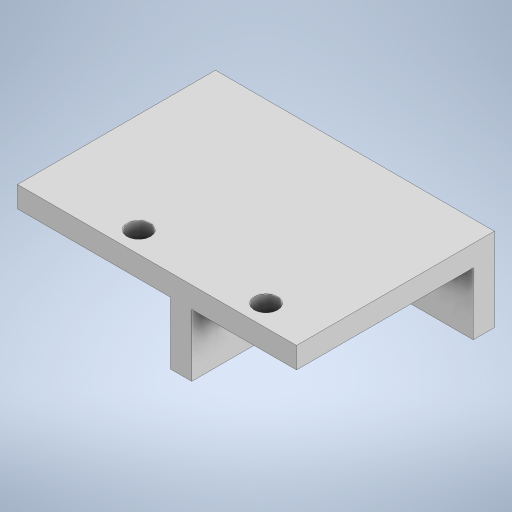
# Autodesk Inventor part: RatPelletBox_v02_holetest
Saved by Autodesk Inventor 2023.5 (Build 275446000, 446)
## iProperties
Created: 2025-06-19
Part Number: RatPelletBox_v02_holetest
Material: Generic
Document SubType Name: Modeling
Designer: Akramilab
Density: 1 g/cm^3
Appearance: Default
Author: Akramilab
Autodesk Inventor part; units mm, degrees
ref_plane "YZ Plane" through (0, 0, 0) normal (1, 0, 0) x (0, 1, 0)
ref_plane "XZ Plane" through (0, 0, 0) normal (0, 1, 0) x (-1, 0, 0)
ref_plane "XY Plane" through (0, 0, 0) normal (0, 0, 1) x (1, 0, 0)
sketch "Sketch1" plane through (0, 0, 0) normal (0, 0, 1) x (1, 0, 0)
  line L0 (-109, -87.5) -> (109, -87.5)
  line L1 (109, -87.5) -> (109, 87.5)
  line L2 (109, 87.5) -> (-109, 87.5)
  line L3 (-109, 87.5) -> (-109, -87.5)
  line L4 (-109, -87.5) -> (109, 87.5) construction
  line L5 (109, -87.5) -> (-109, 87.5) construction
  point P0 (0, 0)
  dimension "d0" = 218
  dimension "d1" = 175
  constraints: 12 end point, 2 midpoint, 2 parallel, 1 horizontal, 1 perpendicular
  measures "d0" distance of L1.end L2.end
  measures "d1" distance of L0.end L1.end
extrude "Extrusion1" add sketch "Sketch1" along normal blind 28
sketch "Sketch2" plane through (0, 0, 28) normal (0, 0, 1) x (1, 0, 0)
  line L0 (-106, 84.5) -> (-66, 84.5)
  line L1 (-66, 84.5) -> (-66, 44.5)
  line L2 (-66, 44.5) -> (-106, 44.5)
  line L3 (-106, 44.5) -> (-106, 84.5)
  line L4 (-106, 84.5) -> (-66, 44.5) construction
  line L5 (-66, 84.5) -> (-106, 44.5) construction
  line L6 (109, 87.5) -> (-109, 87.5) projected
  line L7 (-109, 87.5) -> (-109, -87.5) projected
  line L8 (-63, 84.5) -> (-23, 84.5)
  line L9 (-23, 84.5) -> (-23, 44.5)
  line L10 (-23, 44.5) -> (-63, 44.5)
  line L11 (-63, 44.5) -> (-63, 84.5)
  line L12 (-63, 84.5) -> (-23, 44.5) construction
  line L13 (-23, 84.5) -> (-63, 44.5) construction
  line L14 (-20, 84.5) -> (20, 84.5)
  line L15 (20, 84.5) -> (20, 44.5)
  line L16 (20, 44.5) -> (-20, 44.5)
  line L17 (-20, 44.5) -> (-20, 84.5)
  line L18 (-20, 84.5) -> (20, 44.5) construction
  line L19 (20, 84.5) -> (-20, 44.5) construction
  line L20 (23, 84.5) -> (63, 84.5)
  line L21 (63, 84.5) -> (63, 44.5)
  line L22 (63, 44.5) -> (23, 44.5)
  line L23 (23, 44.5) -> (23, 84.5)
  line L24 (23, 84.5) -> (63, 44.5) construction
  line L25 (63, 84.5) -> (23, 44.5) construction
  line L26 (66, 84.5) -> (106, 84.5)
  line L27 (106, 84.5) -> (106, 44.5)
  line L28 (106, 44.5) -> (66, 44.5)
  line L29 (66, 44.5) -> (66, 84.5)
  line L30 (66, 84.5) -> (106, 44.5) construction
  line L31 (106, 84.5) -> (66, 44.5) construction
  line L32 (-106, 41.5) -> (-66, 41.5)
  line L33 (-66, 41.5) -> (-66, 1.5)
  line L34 (-66, 1.5) -> (-106, 1.5)
  line L35 (-106, 1.5) -> (-106, 41.5)
  line L36 (-106, 41.5) -> (-66, 1.5) construction
  line L37 (-66, 41.5) -> (-106, 1.5) construction
  line L38 (-63, 41.5) -> (-23, 41.5)
  line L39 (-23, 41.5) -> (-23, 1.5)
  line L40 (-23, 1.5) -> (-63, 1.5)
  line L41 (-63, 1.5) -> (-63, 41.5)
  line L42 (-63, 41.5) -> (-23, 1.5) construction
  line L43 (-23, 41.5) -> (-63, 1.5) construction
  line L44 (-20, 41.5) -> (20, 41.5)
  line L45 (20, 41.5) -> (20, 1.5)
  line L46 (20, 1.5) -> (-20, 1.5)
  line L47 (-20, 1.5) -> (-20, 41.5)
  line L48 (-20, 41.5) -> (20, 1.5) construction
  line L49 (20, 41.5) -> (-20, 1.5) construction
  line L50 (23, 41.5) -> (63, 41.5)
  line L51 (63, 41.5) -> (63, 1.5)
  line L52 (63, 1.5) -> (23, 1.5)
  line L53 (23, 1.5) -> (23, 41.5)
  line L54 (23, 41.5) -> (63, 1.5) construction
  line L55 (63, 41.5) -> (23, 1.5) construction
  line L56 (66, 41.5) -> (106, 41.5)
  line L57 (106, 41.5) -> (106, 1.5)
  line L58 (106, 1.5) -> (66, 1.5)
  line L59 (66, 1.5) -> (66, 41.5)
  line L60 (66, 41.5) -> (106, 1.5) construction
  line L61 (106, 41.5) -> (66, 1.5) construction
  line L62 (-106, -1.5) -> (-66, -1.5)
  line L63 (-66, -1.5) -> (-66, -41.5)
  line L64 (-66, -41.5) -> (-106, -41.5)
  line L65 (-106, -41.5) -> (-106, -1.5)
  line L66 (-106, -1.5) -> (-66, -41.5) construction
  line L67 (-66, -1.5) -> (-106, -41.5) construction
  line L68 (-63, -1.5) -> (-23, -1.5)
  line L69 (-23, -1.5) -> (-23, -41.5)
  line L70 (-23, -41.5) -> (-63, -41.5)
  line L71 (-63, -41.5) -> (-63, -1.5)
  line L72 (-63, -1.5) -> (-23, -41.5) construction
  line L73 (-23, -1.5) -> (-63, -41.5) construction
  line L74 (-20, -1.5) -> (20, -1.5)
  line L75 (20, -1.5) -> (20, -41.5)
  line L76 (20, -41.5) -> (-20, -41.5)
  line L77 (-20, -41.5) -> (-20, -1.5)
  line L78 (-20, -1.5) -> (20, -41.5) construction
  line L79 (20, -1.5) -> (-20, -41.5) construction
  line L80 (23, -1.5) -> (63, -1.5)
  line L81 (63, -1.5) -> (63, -41.5)
  line L82 (63, -41.5) -> (23, -41.5)
  line L83 (23, -41.5) -> (23, -1.5)
  line L84 (23, -1.5) -> (63, -41.5) construction
  line L85 (63, -1.5) -> (23, -41.5) construction
  line L86 (66, -1.5) -> (106, -1.5)
  line L87 (106, -1.5) -> (106, -41.5)
  line L88 (106, -41.5) -> (66, -41.5)
  line L89 (66, -41.5) -> (66, -1.5)
  line L90 (66, -1.5) -> (106, -41.5) construction
  line L91 (106, -1.5) -> (66, -41.5) construction
  line L92 (-106, -44.5) -> (-66, -44.5)
  line L93 (-66, -44.5) -> (-66, -84.5)
  line L94 (-66, -84.5) -> (-106, -84.5)
  line L95 (-106, -84.5) -> (-106, -44.5)
  line L96 (-106, -44.5) -> (-66, -84.5) construction
  line L97 (-66, -44.5) -> (-106, -84.5) construction
  line L98 (-63, -44.5) -> (-23, -44.5)
  line L99 (-23, -44.5) -> (-23, -84.5)
  line L100 (-23, -84.5) -> (-63, -84.5)
  line L101 (-63, -84.5) -> (-63, -44.5)
  line L102 (-63, -44.5) -> (-23, -84.5) construction
  line L103 (-23, -44.5) -> (-63, -84.5) construction
  line L104 (-20, -44.5) -> (20, -44.5)
  line L105 (20, -44.5) -> (20, -84.5)
  line L106 (20, -84.5) -> (-20, -84.5)
  line L107 (-20, -84.5) -> (-20, -44.5)
  line L108 (-20, -44.5) -> (20, -84.5) construction
  line L109 (20, -44.5) -> (-20, -84.5) construction
  line L110 (23, -44.5) -> (63, -44.5)
  line L111 (63, -44.5) -> (63, -84.5)
  line L112 (63, -84.5) -> (23, -84.5)
  line L113 (23, -84.5) -> (23, -44.5)
  line L114 (23, -44.5) -> (63, -84.5) construction
  line L115 (63, -44.5) -> (23, -84.5) construction
  line L116 (66, -44.5) -> (106, -44.5)
  line L117 (106, -44.5) -> (106, -84.5)
  line L118 (106, -84.5) -> (66, -84.5)
  line L119 (66, -84.5) -> (66, -44.5)
  line L120 (66, -44.5) -> (106, -84.5) construction
  line L121 (106, -44.5) -> (66, -84.5) construction
  point P0 (0, 0)
  point P1 (-86, 64.5)
  point P2 (-43, 64.5)
  point P3 (0, 64.5)
  point P4 (43, 64.5)
  point P5 (86, 64.5)
  point P6 (-86, 21.5)
  point P7 (-43, 21.5)
  point P8 (0, 21.5)
  point P9 (43, 21.5)
  point P10 (86, 21.5)
  point P11 (-86, -21.5)
  point P12 (-43, -21.5)
  point P13 (0, -21.5)
  point P14 (43, -21.5)
  point P15 (86, -21.5)
  point P16 (-86, -64.5)
  point P17 (-43, -64.5)
  point P18 (0, -64.5)
  point P19 (43, -64.5)
  point P20 (86, -64.5)
  dimension "d4" = 40
  dimension "d5" = 3
  dimension "d6" = 3
  dimension "d7" = 40
  dimension "d10" = 43
  dimension "d13" = 43
  constraints: 240 end point, 2 collinear, 2 horizontal, 2 midpoint, 2 parallel, 1 perpendicular, 1 vertical, 207 other
  measures "d4" distance of L0.start L0.end
  measures "d5" distance between parallel lines of L6 L0
  measures "d6" distance between parallel lines of L7 L3
  measures "d7" distance of L0.end L1.end
  measures "d10" distance of L0.start L8.start
  measures "d13" distance of L0.start L32.start
extrude "Extrusion2" cut sketch "Sketch2" against normal blind 25
sketch "Sketch3" plane through (-109, 87.5, 0) normal (0, 1, 0) x (1, 0, 0)
  line L0 (46, -28) -> (46, -3) construction
  line L1 (43, -28) -> (43, -3) construction
  line L2 (43, -28) -> (43, -3) projected
  line L3 (43, -25) -> (46, -25) construction
  line L4 (46, -28) -> (46, -3) projected
  line L5 (218, -28) -> (0, -28) projected
  circle A0 centre (53.5, -25) radius 1.65
  circle A1 centre (35.5, -25) radius 1.65
  line L6 (172, -28) -> (172, -3) construction
  line L7 (175, -28) -> (175, -3) construction
  line L8 (172, -28) -> (172, -3) projected
  line L9 (172, -25) -> (175, -25) construction
  circle A2 centre (182.5, -25) radius 1.65
  circle A3 centre (164.5, -25) radius 1.65
  point P0 (109, 0)
  point P1 (44.5, -25)
  point P2 (173.5, -25)
  dimension "d20" = 3
  dimension "d21" = 3.3
  dimension "d22" = 9
  dimension "d23" = 3.3
  dimension "d24" = 9
  dimension "d25" = 3.3
  dimension "d27" = 9
  dimension "d30" = 3
  dimension "d31" = 3.3
  dimension "d32" = 9
  constraints: 7 point on line, 4 centre point, 4 end point, 2 midpoint, 2 perpendicular
  measures "d20" distance from line of L5 point (44.5, -25)
  measures "d21" diameter of A0
  measures "d22" distance of A0.centre point (44.5, -25)
  measures "d23" diameter of A1
  measures "d24" distance of A1.centre point (44.5, -25)
  measures "d25" diameter of A2
  measures "d27" distance of A2.centre point (173.5, -25)
  measures "d30" distance from line of L5 point (173.5, -25)
  measures "d31" diameter of A3
  measures "d32" distance of point (173.5, -25) A3.centre
extrude "Extrusion3" cut sketch "Sketch3" against normal blind 10
sketch "Sketch4" plane through (0, 0, 0) normal (0, 0, -1) x (-1, 0, 0)
  line L0 (-109, 87.5) -> (109, 87.5) projected
  line L1 (48.1771, 87.5) -> (-137.115, 87.5)
  line L2 (-137.115, 87.5) -> (-137.115, -97.6556)
  line L3 (-137.115, -97.6556) -> (48.1771, -97.6556)
  line L4 (48.1771, -97.6556) -> (48.1771, 87.5)
  line L5 (153.7374, -115.3645) -> (-15.4329, -115.3645)
  line L6 (-15.4329, -115.3645) -> (-15.4329, 75.6885)
  line L7 (-15.4329, 75.6885) -> (153.7374, 75.6885)
  line L8 (153.7374, 75.6885) -> (153.7374, -115.3645)
  line L9 (153.7374, 38.7258) -> (87.6444, 38.7258)
  line L10 (87.6444, 38.7258) -> (87.6444, 105.9246)
  line L11 (87.6444, 105.9246) -> (153.7374, 105.9246)
  line L12 (153.7374, 105.9246) -> (153.7374, 38.7258)
  point P0 (0, 0)
  point P1 (87.6444, 75.6885)
  point P2 (48.1771, 75.6885)
  point P3 (-15.4329, -97.6556)
  point P4 (153.7374, 75.6885)
  constraints: 24 end point, 6 parallel, 3 horizontal, 3 perpendicular, 2 point on line
extrude "Extrusion4" cut sketch "Sketch4" against normal through all contours L0 L4 L7 L6 L3 L2 L1 | L10 L11 L12 L7 | L7 L10 L9 L8 L5 L6 L3 L4 | L4 L3 L6 L7 | L7 L8 L9 L10
equation "\"d0\" = box_length"
equation "\"d1\" = box_width"
equation "\"d2\" = hole_height + wall"
equation "\"d4\" = hole"
equation "\"d5\" = wall"
equation "\"d6\" = wall"
equation "\"d7\" = hole"
equation "\"d10\" = hole + wall"
equation "\"d13\" = hole + wall"
equation "\"d16\" = hole_height"
equation "\"d23\" = d21"
equation "\"d24\" = d22"
equation "\"d25\" = d21"
equation "\"d27\" = d22"
equation "\"d31\" = d25"
equation "\"d32\" = d27"
equation "\"hole\" = 40"
equation "\"wall\" = 3"
equation "\"hole_height\" = 25"
equation "\"box_length\" = 218"
equation "\"box_width\" = 175"
body "Solid1"
